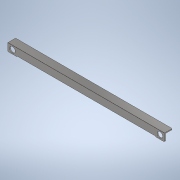
# Autodesk Inventor part: angulo_caja_calor
Saved by Autodesk Inventor 2021 (Build 250183000, 183)
## iProperties
Created: 2021-04-15
Part Number: angulo_caja_calor
Material: Acero inoxidable
Document SubType Name: Modeling
Designer: Leonardo Fabio Mercado Benítez
Density: 8 g/cm^3
Appearance: Semipulido
Author: Leonardo Fabio Mercado Benítez
Autodesk Inventor part; units mm, degrees
ref_plane "YZ Plane" through (0, 0, 0) normal (1, 0, 0) x (0, 1, 0)
ref_plane "XZ Plane" through (0, 0, 0) normal (0, 1, 0) x (-1, 0, 0)
ref_plane "XY Plane" through (0, 0, 0) normal (0, 0, 1) x (1, 0, 0)
sketch "Boceto1" plane through (0, 0, 0) normal (1, 0, 0) x (0, 1, 0)
  line L0 (0, -0.3) -> (0, -25.4)
  line L1 (-0.3, 0) -> (-25.4, 0)
  arc A0 (0, -0.3) -> (-0.3, 0) centre (-0.3, -0.3) ccw
  line L2 (-25.4, 0) -> (-25.4, -3.175)
  line L3 (0, -25.4) -> (-3.175, -25.4)
  line L4 (-3.175, -25.4) -> (-3.175, -3.475)
  line L5 (-3.475, -3.175) -> (-25.4, -3.175)
  arc A1 (-3.175, -3.475) -> (-3.475, -3.175) centre (-3.475, -3.475) ccw
  point P0 (0, 0)
  dimension "d0" = 25.4
  dimension "d1" = 25.4
  dimension "d2" = 0.3
  dimension "d3" = 3.175
  dimension "d4" = 3.175
  dimension "d5" = 0.3
  constraints: 12 end point, 4 point on circle, 4 tangent, 3 vertical, 2 centre point, 2 horizontal, 2 point on line, 1 perpendicular
  measures "d0" distance of point (0, 0) L0.end
  measures "d1" distance of point (0, 0) L1.end
  measures "d2" radius of A0
  measures "d3" distance of L1.end L2.end
  measures "d4" distance of L0.end L3.end
  measures "d5" radius of A1
extrude "Extrusión1" add sketch "Boceto1" along normal blind 515
fillet "Empalme1" radius 2 4 edges at (515, -25.4, -1.5875) (515, -1.5875, -25.4) (0, -25.4, -1.5875) (0, -1.5875, -25.4)
sketch "Boceto3" plane through (0, -0.3, 0) normal (0, 0, 1) x (1, 0, 0)
  line L0 (0, 0) -> (515, 0) construction
  line L1 (257.5, 0) -> (257.5, -25.1) construction
  line L2 (2, -25.1) -> (513, -25.1) construction
  line L3 (257.5, -12.55) -> (500, -12.55) construction
  line L4 (257.5, -12.55) -> (15, -12.55) construction
  circle A0 centre (15, -12.55) radius 9.4375
  circle A1 centre (500, -12.55) radius 9.4375
  dimension "d11" = 242.5
  dimension "d12" = 242.5
  dimension "d13" = 18.875
  dimension "d16" = 18.875
  constraints: 6 end point, 3 midpoint, 2 centre point, 2 horizontal, 1 coincident
  measures "d11" distance of L3.start L3.end
  measures "d12" distance of L3.start L4.end
  measures "d13" diameter of A0
  measures "d16" diameter of A1
extrude "Extrusión2" cut sketch "Boceto3" against normal up to surface (3.175 mm away)
sketch "Boceto4" plane through (0, -0.3, 0) normal (0, 0, 1) x (1, 0, 0)
  arc A0 (13.9157, -3.175) -> (16.0843, -3.175) centre (15, -12.55) ccw projected
  line L0 (2, -25.1) -> (513, -25.1) construction
  line L1 (30, -23.1) -> (30, 0) construction
  line L2 (0, 0) -> (515, 0) construction
  line L3 (28, -25.1) -> (2, -25.1) construction
  arc A1 (28, -25.1) -> (30, -23.1) centre (28, -23.1) ccw
  circle A2 centre (500, -12.55) radius 9.4375 construction
  line L4 (515, -23.1) -> (515, -3.175) construction
  line L5 (485, -23.1) -> (485, 0) construction
  line L6 (487, -25.1) -> (513, -25.1) construction
  arc A3 (485, -23.1) -> (487, -25.1) centre (487, -23.1) ccw
  line L7 (485, -23.1) -> (30, -23.1)
  line L8 (28, -25.1) -> (487, -25.1)
  point P0 (0, 0.3)
  point P1 (30, -25.1)
  point P2 (485, -25.1)
  dimension "d20" = 2
  dimension "d23" = 2
  constraints: 12 end point, 8 point on line, 4 point on circle, 4 tangent, 3 collinear, 2 centre point, 1 perpendicular, 1 vertical
  measures "d20" radius of A1
  measures "d23" radius of A3
extrude "Extrusión3" cut sketch "Boceto4" against normal up to surface (3.175 mm away)
